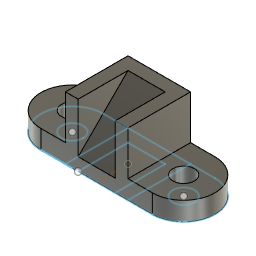
Piece-2 v4 (Autodesk Fusion 360 design; units mm, degrees)
Autodesk Fusion 360 part; units mm, degrees
sketch "Base" plane through (0, 0, 0) normal (0, 0, 1) x (1, 0, 0)
  line L0 (57.1094, -32.1835) -> (-56.8906, -32.1835)
  line L1 (-56.8906, 31.8165) -> (57.1094, 31.8165)
  circle A0 centre (-56.8906, -0.1835) radius 11
  circle A1 centre (57.1094, -0.1835) radius 11
  arc A2 (57.1094, -32.1835) -> (57.1094, 31.8165) centre (57.1094, -0.1835) ccw
  arc A3 (-56.8906, 31.8165) -> (-56.8906, -32.1835) centre (-56.8906, -0.1835) ccw
  line L2 (-31.8906, 31.8165) -> (-31.8906, -32.1835)
  line L3 (32.1094, 31.8165) -> (32.1094, -32.1835)
  line L4 (0.1094, 31.8165) -> (0.1094, -32.1835) construction
  line L5 (19.1094, 18.8165) -> (19.1094, -32.1835)
  line L6 (-18.8906, 18.8165) -> (-18.8906, -32.1835)
  line L7 (-18.8906, 18.8165) -> (19.1094, 18.8165)
  dimension "d6" = 114
  dimension "d7" = 64
  dimension "d9" = 32
  dimension "d10" = 32
  dimension "d11" = 22
  dimension "d12" = 22
  dimension "d15" = 64
  dimension "d16" = 32
  dimension "d17" = 19
  dimension "d18" = 51
  constraint horizontal L0
  constraint parallel L0 L1
  constraint concentric A0 A3
  constraint concentric A1 A2
  constraint coincident L1 L2.start
  constraint coincident L0 L2.end
  constraint perpendicular L0 L2
  constraint coincident L1 L3.start
  constraint coincident L0 L3.end
  constraint perpendicular L0 L3
  constraint midpoint L1 L4.start
  constraint midpoint L0 L4.end
  constraint perpendicular L0 L4
  constraint coincident L0 L5.end
  constraint perpendicular L0 L5
  constraint symmetric L4 L5.end L6.end
  constraint perpendicular L3 L7
  measures "d6" distance of L1.start L1.end
  measures "d7" distance of L0.end L1.start
  measures "d9" radius of A3
  measures "d10" radius of A2
  measures "d11" diameter of A0
  measures "d12" diameter of A1
  measures "d15" distance of L2 L3
  measures "d16" distance of L3 L4
  measures "d17" distance of L4 L5
  measures "d18" distance of L0 L7
extrude "Extrude3" add sketch "Base" along normal blind 64 contours L0 L1 L2 L3 L5 L6 L7 makes body 1
extrude "Extrude4" add sketch "Base" along normal blind 19 contours L0 L1 A3 L2 bodies 1
extrude "Extrude5" add sketch "Base" along normal blind 19 contours L0 L1 A2 L3 bodies 1
extrude "Extrude6" add sketch "Base" along normal blind 64 separate body contours L0 L5 L6 L7 makes body 2
draft "Draft1" angle 45 neutral plane through (-18.8906, 18.8165, 0) pull (0, -1, 0) 1 faces at (6.4427, 1.8165, 64) on bodies 2
combine "Combine1" operation add target body 2 tool bodies 1
equation "d17 = ( 38 / 2 ) * 1 mm"
named bodies: "Main Body", "Piece-2"
